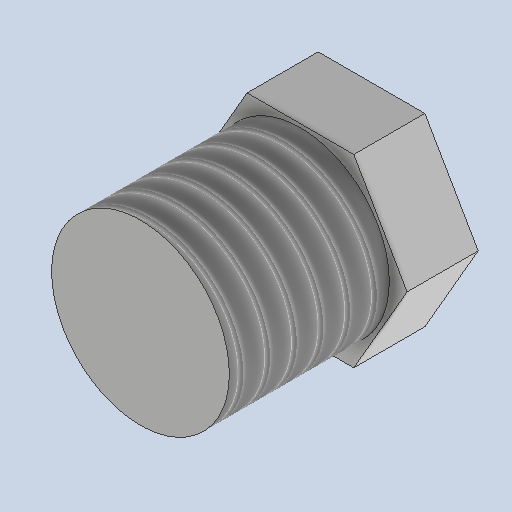
# Autodesk Inventor part: 1157
Saved by Autodesk Inventor 2025.1 (Build 291241000, 241)
## iProperties
Created: 2024-06-07
Part Number: 1157
Material: Generisch
Document SubType Name: Modeling
Designer: ffogue
Density: 1 g/cm^3
Appearance: Vorgabe
Author: ffogue
Autodesk Inventor part; units mm, degrees
ref_plane "YZ Plane" through (0, 0, 0) normal (1, 0, 0) x (0, 1, 0)
ref_plane "XZ Plane" through (0, 0, 0) normal (0, 1, 0) x (-1, 0, 0)
ref_plane "XY Plane" through (0, 0, 0) normal (0, 0, 1) x (1, 0, 0)
sketch "Skizze1" plane through (0, 0, 0) normal (0, 1, 0) x (-1, 0, 0)
  line L0 (6, 0) -> (3, -5.1962)
  line L1 (3, -5.1962) -> (-3, -5.1962)
  line L2 (-3, -5.1962) -> (-6, 0)
  line L3 (-6, 0) -> (-3, 5.1962)
  line L4 (-3, 5.1962) -> (3, 5.1962)
  line L5 (3, 5.1962) -> (6, 0)
  circle A0 centre (0, 0) radius 5
  dimension "d0" = 12
  dimension "d1" = 10
  constraints: 12 end point, 2 coincident, 1 centre point, 13 other
  measures "d0" distance of L2.end L0.start
  measures "d1" diameter of A0
extrude "Extrusion1" add sketch "Skizze1" along normal blind 4
sketch "Skizze2" plane through (0, 4, 0) normal (0, 1, 0) x (1, 0, 0)
  circle A0 centre (0, 0) radius 5
  constraints: 1 centre point, 1 coincident
extrude "Extrusion2" add sketch "Skizze2" against normal blind 13
thread "Gewinde1" size "M10x1.5" class "6g" standard "ISO Metric profile" length 9
